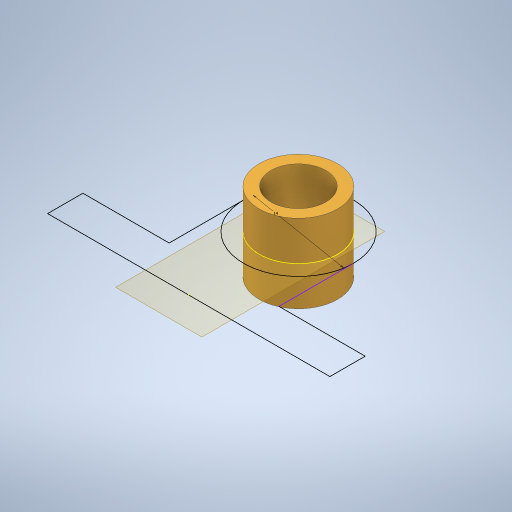
# Autodesk Inventor part: Part1
Saved by Autodesk Inventor 2024.2 (Build 282272000, 272)
## iProperties
Created: 2024-10-24
Part Number: Part1
Material: Generic
Document SubType Name: Modeling
Designer: Precisión-05
Density: 1 g/cm^3
Appearance: Chrome - Polished
Author: Precisión-05
Autodesk Inventor part; units mm, degrees
ref_plane "YZ Plane" through (0, 0, 0) normal (1, 0, 0) x (0, 1, 0)
ref_plane "XZ Plane" through (0, 0, 0) normal (0, 1, 0) x (-1, 0, 0)
sketch "Sketch1" plane through (0, 0, 0) normal (0, 0, 1) x (1, 0, 0)
  line L0 (-25, 0) -> (25, 0) construction
  line L1 (0, 25) -> (0, -25) construction
  line L2 (0, 0) -> (-18, 0)
  line L3 (-18, 0) -> (-18, 4.5)
  line L4 (0, 0) -> (0, 14)
  arc A0 (7, 14) -> (-7, 14) centre (0, 14) ccw
  line L5 (-18, 4.5) -> (-10, 4.5)
  line L6 (-7, 7.5) -> (-7, 14)
  line L7 (0, 0) -> (18, 0)
  line L8 (18, 0) -> (18, 4.5)
  line L9 (18, 4.5) -> (10, 4.5)
  line L10 (7, 7.5) -> (7, 14)
  arc A1 (-10, 4.5) -> (-7, 7.5) centre (-10, 7.5) ccw
  arc A2 (7, 7.5) -> (10, 4.5) centre (10, 7.5) ccw
  circle A3 centre (0, 14) radius 5
  circle A4 centre (0, 14) radius 3.5
  dimension "d0" = 50
  dimension "d1" = 50
  dimension "d2" = 18
  dimension "d3" = 4.5
  dimension "d4" = 14
  dimension "d5" = 14
  dimension "d6" = 18
  dimension "d7" = 4.5
  dimension "d8" = 3
  dimension "d9" = 10
  dimension "d10" = 7
  constraints: 22 end point, 6 point on circle, 6 tangent, 5 centre point, 4 coincident, 3 parallel, 3 point on line, 2 horizontal, 2 midpoint, 2 perpendicular, 1 equal radius, 1 vertical
  measures "d0" distance of L0.start L0.end
  measures "d1" distance of L1.start L1.end
  measures "d2" distance of L2.start L2.end
  measures "d3" distance of L2.end L3.end
  measures "d4" distance of L2.start L4.end
  measures "d5" diameter of A0
  measures "d6" distance of L2.start L7.end
  measures "d7" distance of L7.end L8.end
  measures "d8" radius of A1
  measures "d9" diameter of A3
  measures "d10" diameter of A4
extrude "Extrusion1" add sketch "Sketch1" along normal mid plane 10 contours A3
ref_plane "Work Plane1" through (0, 0, 0) normal (0, 0, 1) x (1, 0, 0)
sketch "Sketch2" plane through (0, 0, 0) normal (0, 0, 1) x (1, 0, 0)
  circle A0 centre (0, 14) radius 5 projected
  circle A1 centre (0, 14) radius 7
  line L0 (-18, 4.5) -> (-10, 4.5) projected
  line L1 (18, 4.5) -> (10, 4.5) projected
  line L2 (0, 0) -> (18, 0) projected
  line L3 (0, 0) -> (-18, 0) projected
  line L4 (-7, 14) -> (-7, 4.5)
  line L5 (-7, 4.5) -> (-18, 4.5)
  line L6 (-18, 4.5) -> (-18, 0)
  line L7 (-18, 0) -> (18, 0)
  line L8 (18, 0) -> (18, 4.5)
  line L9 (18, 4.5) -> (7, 4.5)
  line L10 (7, 4.5) -> (7, 14)
  dimension "d14" = 14
  constraints: 14 end point, 3 perpendicular, 2 collinear, 2 point on circle, 1 centre point, 1 coincident, 1 point on line, 1 tangent, 1 vertical
  measures "d14" diameter of A1
body "Solid1"
